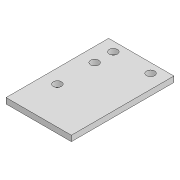
# Autodesk Inventor part: Print_Parts_S_Cap
Saved by Autodesk Inventor 2020 (Build 240168000, 168)
## iProperties
Created: 2020-11-09
Part Number: Print_Parts_S_Cap
Material: 一般
Document SubType Name: Modeling
Designer: kenta iguchi
Density: 1 g/cm^3
Appearance: 既定
Author: kenta iguchi
Autodesk Inventor part; units mm, degrees
ref_plane "YZ Plane" through (0, 0, 0) normal (1, 0, 0) x (0, 1, 0)
ref_plane "XZ Plane" through (0, 0, 0) normal (0, 1, 0) x (-1, 0, 0)
ref_plane "XY Plane" through (0, 0, 0) normal (0, 0, 1) x (1, 0, 0)
sketch "スケッチ43" plane through (0, 0, 0) normal (0, 1, 0) x (-1, 0, 0)
  line L0 (0, 0) -> (35, 0)
  line L1 (35, 0) -> (35, -40)
  line L2 (35, -40) -> (0, -40)
  line L3 (0, -40) -> (0, 0)
  line L4 (35, -23.85) -> (25, -23.85)
  line L5 (25, -23.85) -> (25, -36.15)
  line L6 (25, -36.15) -> (35, -36.15)
  line L7 (35, -36.15) -> (35, -23.85)
  line L8 (25, -36.15) -> (35, -36.15)
  line L9 (35, -36.15) -> (35, -40)
  line L10 (35, -40) -> (25, -40)
  line L11 (25, -40) -> (25, -36.15)
  point P0 (25, -30)
  dimension "d198" = 40
  dimension "d200" = 12.3
  dimension "d201" = 10
  dimension "d202" = 10
  dimension "d203" = 25
  constraints: 24 end point, 6 parallel, 3 horizontal, 3 perpendicular, 1 midpoint, 1 point on line
  measures "d198" distance of L0.end L1.end
  measures "d200" distance of L4.end L5.end
  measures "d201" distance of L5.end L6.end
  measures "d202" distance from line of L2 point (25, -30)
  measures "d203" distance from line of point (25, -30) L3
extrude "押し出し34" add sketch "スケッチ43" along normal blind 3
sketch "スケッチ45" plane through (0, 3, 0) normal (0, 1, 0) x (1, 0, 0)
  line L0 (-35, 40) -> (-35, 0) projected
  line L1 (-35, 0) -> (0, 0) projected
  line L2 (0, 0) -> (0, 40) projected
  line L3 (0, 40) -> (-35, 40) projected
  line L4 (0, 0) -> (0, 40) projected
  line L5 (0, 40) -> (-35, 40)
  line L6 (-35, 40) -> (-35, 55)
  line L7 (-35, 55) -> (0, 55)
  line L8 (0, 55) -> (0, 40)
  point P0 (-35, 40)
  dimension "d217" = 15
  constraints: 8 end point, 2 parallel, 1 horizontal, 1 perpendicular, 1 vertical alignment
  measures "d217" distance of L5.end L6.end
extrude "押し出し35" add sketch "スケッチ45" against normal up to surface (3 mm away) contours L6 L7 L8 L3
sketch "スケッチ46" plane through (0, 3, 0) normal (0, 1, 0) x (1, 0, 0)
  line L0 (-35, 0) -> (0, 0) projected
  line L1 (0, 0) -> (0, 55) projected
  line L2 (0, 55) -> (-35, 55) projected
  line L3 (-35, 55) -> (-35, 0) projected
  point P0 (-27.5, 20)
  point P1 (-27.5, 40)
  point P2 (-27.5, 50)
  point P3 (-7.5, 50)
  dimension "d220" = 20
  dimension "d223" = 20
  dimension "d224" = 10
  dimension "d233" = 7.5
  constraints: 2 vertical alignment, 1 horizontal alignment
  measures "d220" distance of point (-27.5, 40) point (-27.5, 20)
  measures "d223" distance of point (-27.5, 50) point (-7.5, 50)
  measures "d224" distance of point (-27.5, 50) point (-27.5, 40)
  measures "d233" distance from line of point (-27.5, 50) L3
hole "穴8" at (-27.5, 3, -20) at (-27.5, 3, -40) at (-27.5, 3, -50) at (-7.5, 3, -50) direction (0, -1, 0) diameter 4.4 end through all
